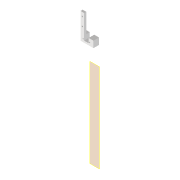
# Autodesk Inventor part: 30_XYTable_Aliexpress_naked_endstopX_adapter
Saved by Autodesk Inventor 2022 (Build 260153000, 153)
## iProperties
Created: 2022-11-01
Part Number: 30_XYTable_Aliexpress_naked_endstopX_adapter
Material: Generisch
Document SubType Name: Modeling
Designer: diederichbenedict
Density: 1 g/cm^3
Appearance: Vorgabe
Author: diederichbenedict
Autodesk Inventor part; units mm, degrees
ref_plane "YZ Plane" through (0, 0, 0) normal (1, 0, 0) x (0, 1, 0)
ref_plane "XZ Plane" through (0, 0, 0) normal (0, 1, 0) x (-1, 0, 0)
ref_plane "XY Plane" through (0, 0, 0) normal (0, 0, 1) x (1, 0, 0)
ref_plane "Arbeitsebene1" through (0, 0, 0) normal (0, 0, 1) x (1, 0, 0)
sketch "Skizze1" plane through (0, 0, 0) normal (0, 0, 1) x (1, 0, 0)
  line L0 (8.8004, 63) -> (20, 63)
  line L1 (20, 63) -> (20, 53)
  line L2 (8.8004, 63) -> (-10, 63)
  line L3 (-10, 63) -> (-10, 53)
  line L4 (-10, 53) -> (20, 53)
  circle A0 centre (-3.9345, 60.036) radius 1.4
  circle A1 centre (11.0655, 60.036) radius 1.4
  line L5 (-10, 63) -> (20, 63)
  line L6 (20, 63) -> (20, 68)
  line L7 (20, 68) -> (-10, 68)
  line L8 (-10, 68) -> (-10, 63)
  point P0 (12.8, 45.75)
  point P1 (12.8, 36.25)
  dimension "d11" = 30
  dimension "d14" = 10
  dimension "d16" = 2.8
  dimension "d17" = 2.8
  dimension "d18" = 15
  dimension "d19" = 0
  dimension "d20" = 5
  constraints: 18 end point, 3 parallel, 2 centre point, 2 horizontal, 2 perpendicular
  measures "d11" distance between parallel lines of L1 L3
  measures "d14" distance between parallel lines of L2 L4
  measures "d16" diameter of A0
  measures "d17" diameter of A1
  measures "d18" distance of A1.centre A0.centre
  measures "d19" vertical distance of A0.centre A1.centre
  measures "d20" distance of L6.end L5.end
extrude "Extrusion1" add sketch "Skizze1" along normal blind 5
sketch "Skizze4" plane through (0, 0, 5) normal (0, 0, 1) x (1, 0, 0)
  line L0 (20, 68) -> (-10, 68) projected
  line L1 (-10, 68) -> (-10, 53) projected
  line L2 (-10, 53) -> (20, 53) projected
  circle A0 centre (-3.9345, 60.036) radius 1.4 projected
  circle A1 centre (11.0655, 60.036) radius 1.4 projected
  line L3 (-1.6845, 57.3969) -> (8.8155, 57.3969)
  line L4 (8.8155, 57.3969) -> (8.8155, 70.8506)
  line L5 (8.8155, 70.8506) -> (-1.6845, 70.8506)
  line L6 (-1.6845, 70.8506) -> (-1.6845, 57.3969)
  line L7 (20, 53) -> (20, 68) projected
  point P0 (0, 0)
  point P1 (8.8155, 68)
  point P2 (-1.6845, 68)
  dimension "d21" = 10.5
  dimension "d22" = 2.25
  constraints: 8 end point, 2 parallel, 1 horizontal, 1 perpendicular
  measures "d21" distance of L5.end L4.end
  measures "d22" distance from line of L6 A0.centre
extrude "Extrusion3" cut sketch "Skizze4" against normal blind 5 contours L4 L3 L6 L0
sketch "Skizze5" plane through (0, 0, 5) normal (0, 0, 1) x (1, 0, 0)
  line L0 (-1.6845, 57.3969) -> (-1.6845, 68) projected
  line L1 (-1.6845, 68) -> (-10, 68) projected
  line L2 (-10, 68) -> (-10, 53) projected
  line L3 (-10, 53) -> (20, 53) projected
  line L4 (20, 53) -> (20, 68) projected
  line L5 (20, 68) -> (8.8155, 68) projected
  line L6 (8.8155, 68) -> (8.8155, 57.3969) projected
  line L7 (8.8155, 57.3969) -> (-1.6845, 57.3969) projected
  circle A0 centre (11.0655, 60.036) radius 1.4 projected
  circle A1 centre (-3.9345, 60.036) radius 1.4 projected
  line L8 (-1.6845, 53) -> (-10, 53)
  line L9 (-10, 53) -> (-10, 113)
  line L10 (-10, 113) -> (-1.6845, 113)
  line L11 (-1.6845, 113) -> (-1.6845, 53)
  circle A2 centre (-5.8422, 84) radius 1.6
  circle A3 centre (-5.8422, 104) radius 1.6
  point P0 (0, 0)
  dimension "d26" = 45
  dimension "d27" = 3.2
  dimension "d28" = 3.2
  dimension "d29" = 20
  dimension "d30" = 16
  constraints: 8 end point, 2 centre point, 2 parallel, 2 point on line, 1 horizontal, 1 perpendicular
  measures "d26" distance between parallel lines of L10 L1
  measures "d27" diameter of A2
  measures "d28" diameter of A3
  measures "d29" distance of A2.centre A3.centre
  measures "d30" distance from line of A2.centre L1
extrude "Extrusion4" add sketch "Skizze5" along normal blind 8
sketch "Skizze6" plane through (0, 0, 5) normal (0, 0, -1) x (-1, 0, 0)
  line L0 (1.6845, 68) -> (10, 68) projected
  line L1 (10, 113) -> (10, 68) projected
  line L2 (1.6845, 113) -> (10, 113) projected
  line L3 (1.6845, 68) -> (1.6845, 113) projected
  circle A0 centre (5.8422, 104) radius 1.6 projected
  circle A1 centre (5.8422, 84) radius 1.6 projected
  line L4 (1.6845, 68) -> (10, 68)
  line L5 (10, 68) -> (10, 113)
  line L6 (10, 113) -> (1.6845, 113)
  line L7 (1.6845, 113) -> (1.6845, 68)
  point P0 (0, 0)
  constraints: 8 end point, 2 parallel, 1 horizontal, 1 perpendicular
extrude "Extrusion5" cut sketch "Skizze6" against normal blind 3
